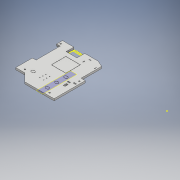
# Autodesk Inventor part: Circuit_handmainboard
Saved by Autodesk Inventor 2018.2 (Build 222227000, 227)
## iProperties
Created: 2018-02-16
Part Number: Circuit_handmainboard
Material: 一般
Document SubType Name: Modeling
Designer: sktom
Density: 1 g/cm^3
Appearance: 既定
Author: sktom
Autodesk Inventor part; units mm, degrees
ref_plane "YZ Plane" through (0, 0, 0) normal (1, 0, 0) x (0, 1, 0)
ref_plane "XZ Plane" through (0, 0, 0) normal (0, 1, 0) x (-1, 0, 0)
ref_plane "XY Plane" through (0, 0, 0) normal (0, 0, 1) x (1, 0, 0)
ref_plane "作業平面1" through (-67.9371, -16.7147, 8.5971) normal (0, 0, -1) x (1, 0, 0)
sketch "スケッチ1" plane through (-67.9371, -16.7147, 8.5971) normal (0, 0, -1) x (1, 0, 0)
  line L0 (13.1301, 23.5542) -> (-11.3844, 23.5542)
  line L1 (-11.3844, 23.5542) -> (-17.9394, 16.9992)
  line L2 (-17.9394, 16.9992) -> (-25.6445, 16.9992)
  line L3 (-25.6445, 16.9992) -> (-25.6445, 2.9992)
  line L4 (-25.6445, 2.9992) -> (-22.5935, 2.9992)
  line L5 (-22.5935, 2.9992) -> (-22.5935, -17.3653)
  line L6 (-22.5935, -17.3653) -> (-25.6833, -17.3653)
  line L7 (-25.6833, -17.3653) -> (-25.6833, -22.3653)
  line L8 (-25.6833, -22.3653) -> (4.3167, -22.3653)
  line L9 (9.5791, -2.734) -> (13.1301, -2.734)
  line L10 (13.1301, -2.734) -> (13.1301, 23.5542)
  line L11 (-25.6445, 19.5692) -> (-19.0435, 19.5692) construction
  line L12 (-25.6445, 19.5692) -> (-25.6445, 17.4992) construction
  line L13 (-25.6445, 17.4992) -> (-18.1465, 17.4992) construction
  line L14 (-18.1465, 17.4992) -> (-11.5915, 24.0542) construction
  line L15 (-11.5915, 24.0542) -> (8.4875, 24.0542) construction
  line L16 (8.4875, 24.0542) -> (8.4875, 26.1242) construction
  line L17 (8.4875, 26.1242) -> (-12.4885, 26.1242) construction
  line L18 (-12.4885, 26.1242) -> (-19.0435, 19.5692) construction
  line L19 (12.2825, 24.0542) -> (14.4905, 24.0542) construction
  line L20 (12.2825, 26.1242) -> (12.2825, 24.0542) construction
  line L21 (12.2825, 24.0542) -> (14.4905, 24.0542) construction
  line L22 (14.4905, 25.4342) -> (14.4905, 24.0542) construction
  line L23 (14.4905, 25.4342) -> (14.4905, 26.1242) construction
  line L24 (14.4905, 26.1242) -> (12.2825, 26.1242) construction
  arc A0 (18.044, 32.4032) -> (16.25, 34.1972) centre (16.25, 32.4032) ccw construction
  line L25 (14.4905, 34.1972) -> (16.25, 34.1972) construction
  line L26 (14.4905, 22.1222) -> (14.4905, 34.1972) construction
  line L27 (14.4905, 22.1222) -> (16.6625, 22.1222) construction
  spline S0 degree 3 poles (16.6625, 22.1222) (16.6025, 24.0843) (16.7566, 25.754) (17.2827, 28.3804) (17.6102, 29.4664) (18.044, 30.5621) knots 0 0 0 0 0.588904 0.588904 1.048143 1.048143 1.048143 1.048143 construction
  line L28 (18.044, 30.5621) -> (18.044, 32.4032) construction
  circle A1 centre (16.25, 32.4032) radius 0.759 construction
  circle A2 centre (6.83, 21.0542) radius 0.55 construction
  circle A3 centre (6.83, 21.0542) radius 1.25 construction
  circle A4 centre (-20.44, 14.4992) radius 1.25 construction
  line L29 (-26.4335, 26.3431) -> (-29.1935, 26.3431) construction
  line L30 (-29.1935, -10.9394) -> (-29.1935, 26.3431) construction
  line L31 (-26.4335, -10.9394) -> (-29.1935, -10.9394) construction
  line L32 (-26.4335, 26.3431) -> (-26.4335, -10.9394) construction
  line L33 (-24.0935, -8.7226) -> (-24.0935, -12.2226) construction
  circle A5 centre (-24.1833, -19.3653) radius 0.55 construction
  circle A6 centre (-24.1833, -19.3653) radius 1.25 construction
  line L34 (9.1301, -21.8653) -> (-26.1833, -21.8653) construction
  line L35 (-26.1833, -21.8653) -> (-26.1833, -22.2455) construction
  spline S1 degree 3 poles (-26.1833, -22.2455) (-26.0411, -22.8107) (-25.8944, -23.3732) (-25.7431, -23.9353) knots 0 0 0 0 1 1 1 1 construction
  line L36 (8.4752, -23.9353) -> (-25.7431, -23.9353) construction
  spline S2 degree 3 poles (8.4752, -23.9353) (8.5807, -23.5922) (8.6886, -23.2482) (8.9069, -22.5597) (9.0189, -22.2107) (9.1301, -21.8653) knots 0 0 0 0 0.496471 0.496471 1 1 1 1 construction
  circle A7 centre (11.1301, 0.266) radius 0.55 construction
  circle A8 centre (11.1301, 0.266) radius 1.25 construction
  line L37 (11.489, 24.0542) -> (11.489, 1.4634) construction
  line L38 (-1.4209, -20.0276) -> (-1.4166, -12.0276) construction
  line L39 (-1.4209, -20.0276) -> (9.5791, -20.0335) construction
  line L40 (9.5834, -12.0335) -> (9.5791, -20.0335) construction
  line L41 (-1.4166, -12.0276) -> (9.5834, -12.0335) construction
  line L42 (8.8105, 9.9742) -> (7.3105, 9.9742) construction
  line L43 (7.3105, 9.9742) -> (7.3105, 7.2742) construction
  line L44 (7.3105, 7.2742) -> (8.8105, 7.2742) construction
  line L45 (8.8105, 7.2742) -> (8.8105, 9.9742) construction
  line L46 (19.5605, 12.1242) -> (6.5605, 12.1242) construction
  line L47 (19.5605, 12.1242) -> (19.5605, 3.1242) construction
  line L48 (19.5605, 3.1242) -> (6.5605, 3.1242) construction
  line L49 (6.5605, 4.8242) -> (6.5605, 3.1242) construction
  line L50 (6.5605, 4.8242) -> (8.2605, 4.8242) construction
  line L51 (8.2605, 4.8242) -> (8.2605, 5.6242) construction
  line L52 (8.2605, 5.6242) -> (6.5605, 5.6242) construction
  line L53 (6.5605, 12.1242) -> (6.5605, 5.6242) construction
  line L54 (11.7605, 4.1242) -> (9.7605, 4.1242) construction
  line L55 (9.7605, 4.1242) -> (9.7605, 3.3242) construction
  line L56 (9.7605, 3.3242) -> (11.7605, 3.3242) construction
  line L57 (11.7605, 3.3242) -> (11.7605, 4.1242) construction
  circle A9 centre (14.5605, 10.1242) radius 0.75 construction
  circle A10 centre (14.5605, 5.1242) radius 0.75 construction
  line L58 (9.5791, -20.0335) -> (4.3167, -22.3653)
  line L59 (9.5791, -20.0335) -> (9.5791, -2.734)
  circle A11 centre (6.83, 21.0542) radius 0.55
  circle A12 centre (-20.44, 14.4992) radius 0.55
  circle A13 centre (11.1301, 0.266) radius 0.55
  circle A14 centre (-24.1833, -19.3653) radius 0.55
  point P0 (67.9371, -16.7147)
  point P1 (9.6055, 25.0467)
  dimension "d0" = 0.5
  dimension "d2" = 0.5
  dimension "d3" = 0.5
  dimension "d4" = 14
  dimension "d5" = 1.5
  dimension "d6" = 2
  dimension "d8" = 0.5
  dimension "d9" = 5
  dimension "d10" = 30
  dimension "d11" = 3
  dimension "d12" = 2
  constraints: 26 end point, 5 perpendicular, 4 centre point, 4 coincident, 4 equal radius, 3 vertical, 2 horizontal, 2 parallel, 1 vertical alignment, 2 other
  measures "d0" distance between parallel lines of L15 L0
  measures "d2" distance between parallel lines of L13 L2
  measures "d3" distance between parallel lines of L14 L1
  measures "d4" distance of L2.end L3.end
  measures "d5" distance between parallel lines of L5 L33
  measures "d6" distance from line of A5.centre L6
  measures "d8" distance between parallel lines of L7 L35
  measures "d9" distance of L6.end L7.end
  measures "d10" distance of L7.end L8.end
  measures "d11" distance from line of A7.centre L9
  measures "d12" distance from line of L10 A7.centre
extrude "押し出し1" add sketch "スケッチ1" along normal blind 1.6
sketch "スケッチ2" plane through (-67.9371, -16.7147, 8.5971) normal (0, 0, 1) x (1, 0, 0)
  line L0 (0.8793, 19.6788) -> (0.8791, 19.9788) projected
  line L1 (0.8791, 19.9788) -> (-0.7209, 19.978) projected
  line L2 (-0.7209, 19.978) -> (-0.7207, 19.678) projected
  line L3 (-0.7207, 19.678) -> (0.8793, 19.6788) projected
  line L4 (-1.5692, 16.8275) -> (-1.5683, 15.2275) projected
  line L5 (-1.5683, 15.2275) -> (-1.2683, 15.2277) projected
  line L6 (-1.2683, 15.2277) -> (-1.2692, 16.8277) projected
  line L7 (-1.2692, 16.8277) -> (-1.5692, 16.8275) projected
  line L8 (8.4317, 15.2329) -> (8.4308, 16.8329) projected
  line L9 (8.4308, 16.8329) -> (8.1308, 16.8327) projected
  line L10 (8.1308, 16.8327) -> (8.1317, 15.2327) projected
  line L11 (8.1317, 15.2327) -> (8.4317, 15.2329) projected
  line L12 (8.8105, -9.9742) -> (8.8105, -7.2742) projected
  line L13 (8.8105, -7.2742) -> (7.3105, -7.2742) projected
  line L14 (7.3105, -7.2742) -> (7.3105, -9.9742) projected
  line L15 (7.3105, -9.9742) -> (8.8105, -9.9742) projected
  line L16 (8.2605, -5.6242) -> (8.2605, -4.8242) projected
  line L17 (8.2605, -4.8242) -> (6.2605, -4.8242) projected
  line L18 (6.2605, -4.8242) -> (6.2605, -5.6242) projected
  line L19 (6.2605, -5.6242) -> (8.2605, -5.6242) projected
  line L20 (11.7605, -4.1242) -> (11.7605, -3.3242) projected
  line L21 (11.7605, -3.3242) -> (9.7605, -3.3242) projected
  line L22 (9.7605, -3.3242) -> (9.7605, -4.1242) projected
  line L23 (9.7605, -4.1242) -> (11.7605, -4.1242) projected
  line L24 (1.9385, -11.6679) -> (2.7385, -11.6675) projected
  arc A0 (2.7385, -11.6675) -> (2.7373, -9.4675) centre (2.7379, -10.5675) ccw projected
  line L25 (2.7373, -9.4675) -> (1.9373, -9.4679) projected
  arc A1 (1.9373, -9.4679) -> (1.9385, -11.6679) centre (1.9379, -10.5679) ccw projected
  line L26 (4.4375, -9.8666) -> (4.4371, -9.1666) projected
  line L27 (4.4375, -9.8666) -> (4.6375, -9.8665) projected
  line L28 (4.6375, -9.8665) -> (4.6371, -9.1665) projected
  line L29 (4.6371, -9.1665) -> (4.4371, -9.1666) projected
  line L30 (4.4386, -11.9666) -> (4.4382, -11.2666) projected
  line L31 (4.6386, -11.9665) -> (4.4386, -11.9666) projected
  line L32 (4.6382, -11.2665) -> (4.6386, -11.9665) projected
  line L33 (4.4382, -11.2666) -> (4.6382, -11.2665) projected
  line L34 (0.2382, -11.2689) -> (0.2386, -11.9689) projected
  line L35 (0.2382, -11.2689) -> (0.0382, -11.269) projected
  line L36 (0.0382, -11.269) -> (0.0386, -11.969) projected
  line L37 (0.0386, -11.969) -> (0.2386, -11.9689) projected
  line L38 (0.2371, -9.1689) -> (0.2375, -9.8689) projected
  line L39 (0.0371, -9.169) -> (0.2371, -9.1689) projected
  line L40 (0.0375, -9.869) -> (0.0371, -9.169) projected
  line L41 (0.2375, -9.8689) -> (0.0375, -9.869) projected
  line L42 (1.9343, -3.8679) -> (2.7343, -3.8675) projected
  arc A2 (2.7343, -3.8675) -> (2.7331, -1.6675) centre (2.7337, -2.7675) ccw projected
  line L43 (2.7331, -1.6675) -> (1.9331, -1.6679) projected
  arc A3 (1.9331, -1.6679) -> (1.9343, -3.8679) centre (1.9337, -2.7679) ccw projected
  line L44 (0.2329, -1.3689) -> (0.2333, -2.0689) projected
  line L45 (0.0329, -1.369) -> (0.2329, -1.3689) projected
  line L46 (0.0333, -2.069) -> (0.0329, -1.369) projected
  line L47 (0.2333, -2.0689) -> (0.0333, -2.069) projected
  line L48 (0.234, -3.4689) -> (0.2344, -4.1689) projected
  line L49 (0.234, -3.4689) -> (0.034, -3.469) projected
  line L50 (0.034, -3.469) -> (0.0344, -4.169) projected
  line L51 (0.0344, -4.169) -> (0.2344, -4.1689) projected
  line L52 (4.4333, -2.0666) -> (4.4329, -1.3666) projected
  line L53 (4.4333, -2.0666) -> (4.6333, -2.0665) projected
  line L54 (4.6333, -2.0665) -> (4.6329, -1.3665) projected
  line L55 (4.6329, -1.3665) -> (4.4329, -1.3666) projected
  line L56 (4.4344, -4.1666) -> (4.434, -3.4666) projected
  line L57 (4.6344, -4.1665) -> (4.4344, -4.1666) projected
  line L58 (4.634, -3.4665) -> (4.6344, -4.1665) projected
  line L59 (4.434, -3.4666) -> (4.634, -3.4665) projected
  line L60 (1.9427, -19.4679) -> (2.7427, -19.4675) projected
  arc A4 (2.7427, -19.4675) -> (2.7415, -17.2675) centre (2.7421, -18.3675) ccw projected
  line L61 (2.7415, -17.2675) -> (1.9415, -17.2679) projected
  arc A5 (1.9415, -17.2679) -> (1.9427, -19.4679) centre (1.9421, -18.3679) ccw projected
  line L62 (4.4417, -17.6666) -> (4.4413, -16.9666) projected
  line L63 (4.4417, -17.6666) -> (4.6417, -17.6665) projected
  line L64 (4.6417, -17.6665) -> (4.6413, -16.9665) projected
  line L65 (4.6413, -16.9665) -> (4.4413, -16.9666) projected
  line L66 (4.4428, -19.7666) -> (4.4424, -19.0666) projected
  line L67 (4.6428, -19.7665) -> (4.4428, -19.7666) projected
  line L68 (4.6424, -19.0665) -> (4.6428, -19.7665) projected
  line L69 (4.4424, -19.0666) -> (4.6424, -19.0665) projected
  line L70 (0.2413, -16.9689) -> (0.2417, -17.6689) projected
  line L71 (0.0413, -16.969) -> (0.2413, -16.9689) projected
  line L72 (0.0417, -17.669) -> (0.0413, -16.969) projected
  line L73 (0.2417, -17.6689) -> (0.0417, -17.669) projected
  line L74 (0.0424, -19.069) -> (0.0428, -19.769) projected
  line L75 (-8.248, -15.9785) -> (-4.748, -15.9766) projected
  line L76 (-8.2489, -14.4285) -> (-8.248, -15.9785) projected
  line L77 (-8.2526, -7.4785) -> (-8.2518, -9.0285) projected
  line L78 (-4.7526, -7.4766) -> (-8.2526, -7.4785) projected
  line L79 (-17.6713, -14.064) -> (-13.4713, -14.0617) projected
  line L80 (-13.4713, -14.0617) -> (-13.473, -10.8617) projected
  line L81 (-13.473, -10.8617) -> (-17.673, -10.864) projected
  line L82 (-17.673, -10.864) -> (-17.6713, -14.064) projected
  line L83 (-13.5213, -14.0117) -> (-14.3713, -14.0122) projected
  line L84 (-14.3713, -14.0122) -> (-13.5217, -13.1617) projected
  line L85 (-13.5217, -13.1617) -> (-13.5213, -14.0117) projected
  line L86 (-16.7713, -14.0135) -> (-17.6213, -14.0139) projected
  line L87 (-17.6213, -14.0139) -> (-17.6217, -13.1639) projected
  line L88 (-17.6217, -13.1639) -> (-16.7713, -14.0135) projected
  line L89 (-14.3729, -10.9122) -> (-13.523, -10.9117) projected
  line L90 (-13.523, -10.9117) -> (-13.5225, -11.7617) projected
  line L91 (-13.5225, -11.7617) -> (-14.3729, -10.9122) projected
  line L92 (-17.6229, -10.9139) -> (-16.7729, -10.9135) projected
  line L93 (-16.7729, -10.9135) -> (-17.6225, -11.7639) projected
  line L94 (-17.6225, -11.7639) -> (-17.6229, -10.9139) projected
  arc A6 (-15.9727, -11.363) -> (-15.9715, -13.563) centre (-15.9721, -12.463) ccw projected
  line L95 (-15.9727, -11.363) -> (-15.1727, -11.3626) projected
  arc A7 (-15.1715, -13.5626) -> (-15.1727, -11.3626) centre (-15.1721, -12.4626) ccw projected
  line L96 (-15.1715, -13.5626) -> (-15.9715, -13.563) projected
  line L97 (-1.5207, 1.0375) -> (-1.5262, 11.2275) projected
  line L98 (-11.7107, 1.032) -> (-1.5207, 1.0375) projected
  line L99 (-11.7162, 11.222) -> (-11.7107, 1.032) projected
  line L100 (-1.5262, 11.2275) -> (-11.7162, 11.222) projected
  line L101 (-0.5201, 0.0381) -> (-12.7101, 0.0315) projected
  line L102 (-0.5267, 12.2281) -> (-0.5201, 0.0381) projected
  line L103 (-12.7167, 12.2215) -> (-0.5267, 12.2281) projected
  line L104 (-12.7101, 0.0315) -> (-12.7167, 12.2215) projected
  point P0 (67.9371, 16.7147)
sketch "スケッチ3" plane through (-67.9371, -16.7147, 6.9971) normal (0, 0, -1) x (-1, 0, 0)
  line L0 (19.1277, -4.5638) -> (3.8877, -4.5555) projected
  line L1 (19.1414, 20.8362) -> (19.1277, -4.5638) projected
  line L2 (3.9014, 20.8445) -> (19.1414, 20.8362) projected
  line L3 (3.8877, -4.5555) -> (3.9014, 20.8445) projected
  circle A0 centre (8.9697, -0.7483) radius 0.51 projected
  circle A1 centre (11.5097, -0.7497) radius 0.51 projected
  circle A2 centre (14.0497, -0.751) radius 0.51 projected
  circle A3 centre (5.1597, -0.7462) radius 0.51 projected
  circle A4 centre (5.1625, 4.3338) radius 0.51 projected
  circle A5 centre (5.1652, 9.4138) radius 0.51 projected
  circle A6 centre (5.1679, 14.4938) radius 0.51 projected
  circle A7 centre (5.1707, 19.5738) radius 0.51 projected
  circle A8 centre (17.8597, -0.7531) radius 0.51 projected
  circle A9 centre (17.8625, 4.3269) radius 0.51 projected
  circle A10 centre (17.8652, 9.4069) radius 0.51 projected
  circle A11 centre (17.8679, 14.4869) radius 0.51 projected
  circle A12 centre (17.8707, 19.5669) radius 0.51 projected
  circle A13 centre (17.8693, 17.0269) radius 0.51 projected
  circle A14 centre (17.8666, 11.9469) radius 0.51 projected
  circle A15 centre (17.8638, 6.8669) radius 0.51 projected
  circle A16 centre (17.8611, 1.7869) radius 0.51 projected
  circle A17 centre (17.8584, -3.2931) radius 0.51 projected
  circle A18 centre (5.1693, 17.0338) radius 0.51 projected
  circle A19 centre (5.1666, 11.9538) radius 0.51 projected
  circle A20 centre (5.1638, 6.8738) radius 0.51 projected
  circle A21 centre (5.1611, 1.7938) radius 0.51 projected
  circle A22 centre (5.1584, -3.2862) radius 0.51 projected
  circle A23 centre (14.0484, -3.291) radius 0.51 projected
  circle A24 centre (11.5084, -3.2897) radius 0.51 projected
  circle A25 centre (8.9684, -3.2883) radius 0.51 projected
  line L4 (20.6136, 6.3654) -> (20.6141, 7.3654) projected
  line L5 (20.6141, 7.3654) -> (19.1141, 7.3662) projected
  line L6 (19.1136, 6.3662) -> (19.1141, 7.3662) projected
  line L7 (19.1136, 6.3662) -> (20.6136, 6.3654) projected
  line L8 (20.6163, 11.4454) -> (20.6168, 12.4454) projected
  line L9 (20.6168, 12.4454) -> (19.1168, 12.4462) projected
  line L10 (19.1163, 11.4462) -> (19.1168, 12.4462) projected
  line L11 (19.1163, 11.4462) -> (20.6163, 11.4454) projected
  line L12 (20.619, 16.5254) -> (20.6196, 17.5254) projected
  line L13 (20.6196, 17.5254) -> (19.1196, 17.5262) projected
  line L14 (19.119, 16.5262) -> (19.1196, 17.5262) projected
  line L15 (19.119, 16.5262) -> (20.619, 16.5254) projected
  line L16 (19.1108, 1.2863) -> (20.6108, 1.2854) projected
  line L17 (20.6108, 1.2854) -> (20.6114, 2.2854) projected
  line L18 (20.6114, 2.2854) -> (19.1114, 2.2862) projected
  line L19 (19.1108, 1.2863) -> (19.1114, 2.2862) projected
  line L20 (19.1108, 1.2863) -> (20.6108, 1.2854) projected
  line L21 (20.6081, -3.7946) -> (20.6086, -2.7946) projected
  line L22 (20.6086, -2.7946) -> (19.1086, -2.7937) projected
  line L23 (19.1081, -3.7937) -> (19.1086, -2.7937) projected
  line L24 (19.1081, -3.7937) -> (20.6081, -3.7946) projected
  line L25 (2.4095, -1.2447) -> (2.41, -0.2447) projected
  line L26 (3.9095, -1.2456) -> (2.4095, -1.2447) projected
  line L27 (3.91, -0.2456) -> (3.9095, -1.2456) projected
  line L28 (2.41, -0.2447) -> (3.91, -0.2456) projected
  line L29 (2.4122, 3.8353) -> (2.4127, 4.8353) projected
  line L30 (3.9122, 3.8344) -> (2.4122, 3.8353) projected
  line L31 (3.9127, 4.8344) -> (3.9122, 3.8344) projected
  line L32 (2.4127, 4.8353) -> (3.9127, 4.8344) projected
  line L33 (2.4149, 8.9153) -> (2.4155, 9.9153) projected
  line L34 (3.9149, 8.9144) -> (2.4149, 8.9153) projected
  line L35 (3.9155, 9.9144) -> (3.9149, 8.9144) projected
  line L36 (2.4155, 9.9153) -> (3.9155, 9.9144) projected
  line L37 (2.4177, 13.9953) -> (2.4182, 14.9953) projected
  line L38 (3.9177, 13.9944) -> (2.4177, 13.9953) projected
  line L39 (3.9182, 14.9944) -> (3.9177, 13.9944) projected
  line L40 (2.4182, 14.9953) -> (3.9182, 14.9944) projected
  line L41 (2.4204, 19.0752) -> (2.4209, 20.0752) projected
  line L42 (3.9204, 19.0744) -> (2.4204, 19.0752) projected
  line L43 (3.9209, 20.0744) -> (3.9204, 19.0744) projected
  line L44 (2.4209, 20.0752) -> (3.9209, 20.0744) projected
  circle A26 centre (8.1017, -9.2284) radius 0.25 projected
  circle A27 centre (8.1003, -11.7284) radius 0.25 projected
  circle A28 centre (8.099, -14.2284) radius 0.25 projected
  circle A29 centre (4.899, -14.2266) radius 0.25 projected
  circle A30 centre (4.9003, -11.7266) radius 0.25 projected
  circle A31 centre (4.9017, -9.2266) radius 0.25 projected
  line L45 (-7.3839, 11.0323) -> (-6.0839, 11.0316) projected
  line L46 (-7.3839, 11.0323) -> (-7.3854, 8.2323) projected
  line L47 (-7.3854, 8.2323) -> (-6.0854, 8.2316) projected
  line L48 (-6.0839, 11.0316) -> (-6.0854, 8.2316) projected
  line L49 (-0.1839, 11.0284) -> (1.1161, 11.0277) projected
  line L50 (-0.1839, 11.0284) -> (-0.1854, 8.2284) projected
  line L51 (-0.1854, 8.2284) -> (1.1146, 8.2277) projected
  line L52 (1.1161, 11.0277) -> (1.1146, 8.2277) projected
  line L53 (-1.7259, 7.4263) -> (-1.7261, 6.9293) projected
  line L54 (-1.7259, 7.4263) -> (-2.0459, 7.4264) projected
  line L55 (-2.0459, 7.4264) -> (-2.0461, 6.9294) projected
  line L56 (-1.7261, 6.9293) -> (-2.0461, 6.9294) projected
  line L57 (-2.9759, 7.4269) -> (-2.9761, 6.9299) projected
  line L58 (-2.9759, 7.4269) -> (-3.2959, 7.4271) projected
  line L59 (-3.2959, 7.4271) -> (-3.2961, 6.9301) projected
  line L60 (-2.9761, 6.9299) -> (-3.2961, 6.9301) projected
  line L61 (-4.2259, 7.4276) -> (-4.2261, 6.9306) projected
  line L62 (-4.2259, 7.4276) -> (-4.5459, 7.4278) projected
  line L63 (-4.5459, 7.4278) -> (-4.5461, 6.9308) projected
  line L64 (-4.2261, 6.9306) -> (-4.5461, 6.9308) projected
  line L65 (-0.1867, 5.8284) -> (1.1133, 5.8277) projected
  line L66 (-0.1867, 5.8284) -> (-0.1882, 3.0284) projected
  line L67 (-0.1882, 3.0284) -> (1.1118, 3.0277) projected
  line L68 (1.1133, 5.8277) -> (1.1118, 3.0277) projected
  line L69 (-7.3867, 5.8323) -> (-6.0867, 5.8316) projected
  line L70 (-7.3867, 5.8323) -> (-7.3882, 3.0323) projected
  line L71 (-7.3882, 3.0323) -> (-6.0882, 3.0316) projected
  line L72 (-6.0867, 5.8316) -> (-6.0882, 3.0316) projected
  line L73 (-4.2287, 2.2276) -> (-4.2289, 1.7306) projected
  line L74 (-4.2287, 2.2276) -> (-4.5487, 2.2278) projected
  line L75 (-4.5487, 2.2278) -> (-4.5489, 1.7308) projected
  line L76 (-4.2289, 1.7306) -> (-4.5489, 1.7308) projected
  line L77 (-2.9787, 2.2269) -> (-2.9789, 1.7299) projected
  line L78 (-2.9787, 2.2269) -> (-3.2987, 2.2271) projected
  line L79 (-3.2987, 2.2271) -> (-3.2989, 1.7301) projected
  line L80 (-2.9789, 1.7299) -> (-3.2989, 1.7301) projected
  line L81 (-1.7287, 2.2263) -> (-1.7289, 1.7293) projected
  line L82 (-1.7287, 2.2263) -> (-2.0487, 2.2264) projected
  line L83 (-2.0487, 2.2264) -> (-2.0489, 1.7294) projected
  line L84 (-1.7289, 1.7293) -> (-2.0489, 1.7294) projected
  line L85 (25.465, -4.935) -> (25.4643, -6.235) projected
  line L86 (25.465, -4.935) -> (22.665, -4.9335) projected
  line L87 (22.665, -4.9335) -> (22.6643, -6.2335) projected
  line L88 (25.4643, -6.235) -> (22.6643, -6.2335) projected
  line L89 (21.8603, -8.093) -> (21.3633, -8.0928) projected
  line L90 (21.8603, -8.093) -> (21.8604, -7.773) projected
  line L91 (21.8604, -7.773) -> (21.3634, -7.7728) projected
  line L92 (21.3633, -8.0928) -> (21.3634, -7.7728) projected
  line L93 (21.8596, -9.343) -> (21.3626, -9.3428) projected
  line L94 (21.8596, -9.343) -> (21.8598, -9.023) projected
  line L95 (21.8598, -9.023) -> (21.3628, -9.0228) projected
  line L96 (21.3626, -9.3428) -> (21.3628, -9.0228) projected
  line L97 (21.8589, -10.593) -> (21.3619, -10.5928) projected
  line L98 (21.8589, -10.593) -> (21.8591, -10.273) projected
  line L99 (21.8591, -10.273) -> (21.3621, -10.2728) projected
  line L100 (21.3619, -10.5928) -> (21.3621, -10.2728) projected
  line L101 (25.4611, -12.135) -> (25.4604, -13.435) projected
  line L102 (25.4611, -12.135) -> (22.6611, -12.1335) projected
  line L103 (22.6611, -12.1335) -> (22.6604, -13.4335) projected
  line L104 (25.4604, -13.435) -> (22.6604, -13.4335) projected
  line L105 (17.869, 16.5269) -> (17.8696, 17.5269) projected
  line L106 (17.8696, 17.5269) -> (20.6196, 17.5254) projected
  line L107 (20.6196, 17.5254) -> (20.619, 16.5254) projected
  line L108 (20.619, 16.5254) -> (17.869, 16.5269) projected
  line L109 (17.8709, 20.0669) -> (17.8704, 19.0669) projected
  line L110 (17.8704, 19.0669) -> (15.1204, 19.0684) projected
  line L111 (15.1204, 19.0684) -> (15.1209, 20.0684) projected
  line L112 (15.1209, 20.0684) -> (17.8709, 20.0669) projected
  line L113 (16.6177, 13.9876) -> (15.1177, 13.9884) projected
  line L114 (17.8682, 14.9869) -> (17.8677, 13.9869) projected
  line L115 (17.8677, 13.9869) -> (15.1177, 13.9884) projected
  line L116 (15.1177, 13.9884) -> (15.1182, 14.9884) projected
  line L117 (15.1182, 14.9884) -> (17.8682, 14.9869) projected
  line L118 (17.8663, 11.4469) -> (17.8668, 12.4469) projected
  line L119 (17.8668, 12.4469) -> (20.6168, 12.4454) projected
  line L120 (20.6168, 12.4454) -> (20.6163, 11.4454) projected
  line L121 (20.6163, 11.4454) -> (17.8663, 11.4469) projected
  line L122 (17.8655, 9.9069) -> (17.8649, 8.9069) projected
  line L123 (17.8649, 8.9069) -> (15.1149, 8.9084) projected
  line L124 (15.1149, 8.9084) -> (15.1155, 9.9084) projected
  line L125 (15.1155, 9.9084) -> (17.8655, 9.9069) projected
  line L126 (17.8636, 6.3669) -> (17.8641, 7.3669) projected
  line L127 (17.8641, 7.3669) -> (20.6141, 7.3654) projected
  line L128 (20.6141, 7.3654) -> (20.6136, 6.3654) projected
  line L129 (20.6136, 6.3654) -> (17.8636, 6.3669) projected
  line L130 (17.8627, 4.8269) -> (17.8622, 3.8269) projected
  line L131 (17.8622, 3.8269) -> (15.1122, 3.8284) projected
  line L132 (15.1122, 3.8284) -> (15.1127, 4.8284) projected
  line L133 (15.1127, 4.8284) -> (17.8627, 4.8269) projected
  line L134 (17.8608, 1.2869) -> (17.8614, 2.2869) projected
  line L135 (17.8614, 2.2869) -> (20.6114, 2.2854) projected
  line L136 (20.6114, 2.2854) -> (20.6108, 1.2854) projected
  line L137 (20.6108, 1.2854) -> (17.8608, 1.2869) projected
  line L138 (17.86, -0.2531) -> (17.8595, -1.2531) projected
  line L139 (17.8595, -1.2531) -> (15.1095, -1.2516) projected
  line L140 (15.1095, -1.2516) -> (15.11, -0.2516) projected
  line L141 (15.11, -0.2516) -> (17.86, -0.2531) projected
  line L142 (17.8581, -3.7931) -> (17.8586, -2.7931) projected
  line L143 (17.8586, -2.7931) -> (20.6086, -2.7946) projected
  line L144 (20.6086, -2.7946) -> (20.6081, -3.7946) projected
  line L145 (20.6081, -3.7946) -> (17.8581, -3.7931) projected
  line L146 (5.1581, -3.7862) -> (5.1586, -2.7862) projected
  line L147 (5.1586, -2.7862) -> (7.9086, -2.7877) projected
  line L148 (7.9086, -2.7877) -> (7.9081, -3.7877) projected
  line L149 (7.9081, -3.7877) -> (5.1581, -3.7862) projected
  line L150 (5.16, -0.2462) -> (5.1595, -1.2462) projected
  line L151 (5.1595, -1.2462) -> (2.4095, -1.2447) projected
  line L152 (2.4095, -1.2447) -> (2.41, -0.2447) projected
  line L153 (2.41, -0.2447) -> (5.16, -0.2462) projected
  line L154 (5.1608, 1.2938) -> (5.1614, 2.2938) projected
  line L155 (5.1614, 2.2938) -> (7.9114, 2.2923) projected
  line L156 (7.9114, 2.2923) -> (7.9108, 1.2923) projected
  line L157 (7.9108, 1.2923) -> (5.1608, 1.2938) projected
  line L158 (5.1709, 20.0738) -> (5.1704, 19.0738) projected
  line L159 (5.1704, 19.0738) -> (2.4204, 19.0752) projected
  line L160 (2.4204, 19.0752) -> (2.4209, 20.0752) projected
  line L161 (2.4209, 20.0752) -> (5.1709, 20.0738) projected
  line L162 (5.169, 16.5338) -> (5.1696, 17.5338) projected
  line L163 (5.1696, 17.5338) -> (7.9196, 17.5323) projected
  line L164 (7.9196, 17.5323) -> (7.919, 16.5323) projected
  line L165 (7.919, 16.5323) -> (5.169, 16.5338) projected
  line L166 (5.1682, 14.9938) -> (5.1677, 13.9938) projected
  line L167 (5.1677, 13.9938) -> (2.4177, 13.9953) projected
  line L168 (2.4177, 13.9953) -> (2.4182, 14.9953) projected
  line L169 (2.4182, 14.9953) -> (5.1682, 14.9938) projected
  line L170 (5.1663, 11.4538) -> (5.1668, 12.4538) projected
  line L171 (5.1668, 12.4538) -> (7.9168, 12.4523) projected
  line L172 (7.9168, 12.4523) -> (7.9163, 11.4523) projected
  line L173 (7.9163, 11.4523) -> (5.1663, 11.4538) projected
  line L174 (5.1655, 9.9138) -> (5.1649, 8.9138) projected
  line L175 (5.1649, 8.9138) -> (2.4149, 8.9153) projected
  line L176 (2.4149, 8.9153) -> (2.4155, 9.9153) projected
  line L177 (2.4155, 9.9153) -> (5.1655, 9.9138) projected
  point P0 (-67.9371, 16.7147)
extrude "押し出し2" cut sketch "スケッチ2" against normal up to next contours L3 L2 L1 L0 | L7 L6 L5 L4 | L11 L10 L9 L8
sketch "スケッチ4" plane through (-67.9371, -16.7147, 8.5971) normal (0, 0, 1) x (1, 0, 0)
  line L0 (7.3105, -7.2742) -> (7.3105, -9.9742) projected
  line L1 (6.2605, -4.8242) -> (6.2605, -5.6242) projected
  line L2 (9.7605, -3.3242) -> (9.7605, -4.1242) projected
  line L3 (8.8105, -9.9742) -> (8.8105, -7.2742) projected
  line L4 (8.2605, -5.6242) -> (8.2605, -4.8242) projected
  line L5 (11.7605, -4.1242) -> (11.7605, -3.3242) projected
  line L6 (7.3105, -9.9742) -> (8.8105, -9.9742)
  line L7 (8.8105, -9.9742) -> (8.8105, -7.2742)
  line L8 (8.8105, -7.2742) -> (7.3105, -7.2742)
  line L9 (7.3105, -7.2742) -> (7.3105, -9.9742)
  line L10 (6.2605, -5.6242) -> (8.2605, -5.6242)
  line L11 (8.2605, -5.6242) -> (8.2605, -4.8242)
  line L12 (8.2605, -4.8242) -> (6.2605, -4.8242)
  line L13 (6.2605, -4.8242) -> (6.2605, -5.6242)
  line L14 (9.7605, -4.1242) -> (11.7605, -4.1242)
  line L15 (11.7605, -4.1242) -> (11.7605, -3.3242)
  line L16 (11.7605, -3.3242) -> (9.7605, -3.3242)
  line L17 (9.7605, -3.3242) -> (9.7605, -4.1242)
  point P0 (67.9371, 16.7147)
  constraints: 24 end point, 6 parallel, 3 horizontal, 3 perpendicular
extrude "押し出し3" cut sketch "スケッチ4" against normal blind 1.6
sketch "スケッチ5" plane through (-67.9371, -16.7147, 8.5971) normal (0, 0, 1) x (1, 0, 0)
  arc A0 (1.9331, -1.6679) -> (1.9343, -3.8679) centre (1.9337, -2.7679) ccw projected
  line L0 (2.7331, -1.6675) -> (1.9331, -1.6679) projected
  arc A1 (2.7343, -3.8675) -> (2.7331, -1.6675) centre (2.7337, -2.7675) ccw projected
  line L1 (1.9343, -3.8679) -> (2.7343, -3.8675) projected
  line L2 (2.7373, -9.4675) -> (1.9373, -9.4679) projected
  arc A2 (1.9373, -9.4679) -> (1.9385, -11.6679) centre (1.9379, -10.5679) ccw projected
  line L3 (1.9385, -11.6679) -> (2.7385, -11.6675) projected
  arc A3 (2.7385, -11.6675) -> (2.7373, -9.4675) centre (2.7379, -10.5675) ccw projected
  line L4 (2.7415, -17.2675) -> (1.9415, -17.2679) projected
  arc A4 (1.9415, -17.2679) -> (1.9427, -19.4679) centre (1.9421, -18.3679) ccw projected
  line L5 (1.9427, -19.4679) -> (2.7427, -19.4675) projected
  arc A5 (2.7427, -19.4675) -> (2.7415, -17.2675) centre (2.7421, -18.3675) ccw projected
  arc A6 (-15.9727, -11.363) -> (-15.9715, -13.563) centre (-15.9721, -12.463) ccw projected
  line L6 (-15.9727, -11.363) -> (-15.1727, -11.3626) projected
  arc A7 (-15.1715, -13.5626) -> (-15.1727, -11.3626) centre (-15.1721, -12.4626) ccw projected
  line L7 (-15.1715, -13.5626) -> (-15.9715, -13.563) projected
  point P0 (67.9371, 16.7147)
extrude "押し出し4" cut sketch "スケッチ5" against normal blind 0.1
sketch "スケッチ6" plane through (-67.9371, -16.7147, 8.5971) normal (0, 0, 1) x (1, 0, 0)
  line L0 (-12.7101, 0.0315) -> (-12.7167, 12.2215) projected
  line L1 (-12.7167, 12.2215) -> (-0.5267, 12.2281) projected
  line L2 (-0.5267, 12.2281) -> (-0.5201, 0.0381) projected
  line L3 (-0.5201, 0.0381) -> (-12.7101, 0.0315) projected
  point P0 (67.9371, 16.7147)
extrude "押し出し5" cut sketch "スケッチ6" against normal blind 0.1
sketch "スケッチ7" plane through (-67.9371, -16.7147, 6.9971) normal (0, 0, -1) x (-1, 0, 0)
  circle A0 centre (4.899, -14.2266) radius 0.25 projected
  circle A1 centre (8.099, -14.2284) radius 0.25 projected
  circle A2 centre (8.1003, -11.7284) radius 0.25 projected
  circle A3 centre (4.9003, -11.7266) radius 0.25 projected
  circle A4 centre (4.9017, -9.2266) radius 0.25 projected
  circle A5 centre (8.1017, -9.2284) radius 0.25 projected
  point P0 (-67.9371, 16.7147)
extrude "押し出し6" cut sketch "スケッチ3" against normal up to next contours A26 | A27 | A28 | A29 | A30 | A31
sketch "スケッチ8" plane through (-67.9371, -16.7147, 6.9971) normal (0, 0, -1) x (-1, 0, 0)
  line L0 (22.665, -4.9335) -> (22.6643, -6.2335) projected
  line L1 (25.4643, -6.235) -> (22.6643, -6.2335) projected
  line L2 (25.465, -4.935) -> (22.665, -4.9335) projected
  line L3 (25.465, -4.935) -> (25.4643, -6.235) projected
  line L4 (25.4611, -12.135) -> (22.6611, -12.1335) projected
  line L5 (22.6611, -12.1335) -> (22.6604, -13.4335) projected
  line L6 (25.4604, -13.435) -> (22.6604, -13.4335) projected
  line L7 (25.4611, -12.135) -> (25.4604, -13.435) projected
  line L8 (21.8591, -10.273) -> (21.3621, -10.2728) projected
  line L9 (21.3619, -10.5928) -> (21.3621, -10.2728) projected
  line L10 (21.8589, -10.593) -> (21.3619, -10.5928) projected
  line L11 (21.8589, -10.593) -> (21.8591, -10.273) projected
  line L12 (21.3626, -9.3428) -> (21.3628, -9.0228) projected
  line L13 (21.8596, -9.343) -> (21.3626, -9.3428) projected
  line L14 (21.8598, -9.023) -> (21.3628, -9.0228) projected
  line L15 (21.8596, -9.343) -> (21.8598, -9.023) projected
  line L16 (21.8603, -8.093) -> (21.3633, -8.0928) projected
  line L17 (21.3633, -8.0928) -> (21.3634, -7.7728) projected
  line L18 (21.8604, -7.773) -> (21.3634, -7.7728) projected
  line L19 (21.8603, -8.093) -> (21.8604, -7.773) projected
  line L20 (-7.3867, 5.8323) -> (-6.0867, 5.8316) projected
  line L21 (-7.3867, 5.8323) -> (-7.3882, 3.0323) projected
  line L22 (-7.3882, 3.0323) -> (-6.0882, 3.0316) projected
  line L23 (-6.0867, 5.8316) -> (-6.0882, 3.0316) projected
  line L24 (-0.1867, 5.8284) -> (-0.1882, 3.0284) projected
  line L25 (-0.1882, 3.0284) -> (1.1118, 3.0277) projected
  line L26 (1.1133, 5.8277) -> (1.1118, 3.0277) projected
  line L27 (-0.1867, 5.8284) -> (1.1133, 5.8277) projected
  line L28 (-1.7287, 2.2263) -> (-1.7289, 1.7293) projected
  line L29 (-1.7287, 2.2263) -> (-2.0487, 2.2264) projected
  line L30 (-2.0487, 2.2264) -> (-2.0489, 1.7294) projected
  line L31 (-1.7289, 1.7293) -> (-2.0489, 1.7294) projected
  line L32 (-2.9789, 1.7299) -> (-3.2989, 1.7301) projected
  line L33 (-2.9787, 2.2269) -> (-2.9789, 1.7299) projected
  line L34 (-2.9787, 2.2269) -> (-3.2987, 2.2271) projected
  line L35 (-3.2987, 2.2271) -> (-3.2989, 1.7301) projected
  line L36 (-4.2287, 2.2276) -> (-4.2289, 1.7306) projected
  line L37 (-4.5487, 2.2278) -> (-4.5489, 1.7308) projected
  line L38 (-4.2287, 2.2276) -> (-4.5487, 2.2278) projected
  line L39 (-4.2289, 1.7306) -> (-4.5489, 1.7308) projected
  line L40 (-7.3854, 8.2323) -> (-6.0854, 8.2316) projected
  line L41 (-6.0839, 11.0316) -> (-6.0854, 8.2316) projected
  line L42 (-7.3839, 11.0323) -> (-6.0839, 11.0316) projected
  line L43 (-7.3839, 11.0323) -> (-7.3854, 8.2323) projected
  line L44 (-4.5459, 7.4278) -> (-4.5461, 6.9308) projected
  line L45 (-4.2259, 7.4276) -> (-4.5459, 7.4278) projected
  line L46 (-4.2259, 7.4276) -> (-4.2261, 6.9306) projected
  line L47 (-4.2261, 6.9306) -> (-4.5461, 6.9308) projected
  line L48 (-3.2959, 7.4271) -> (-3.2961, 6.9301) projected
  line L49 (-2.9759, 7.4269) -> (-3.2959, 7.4271) projected
  line L50 (-2.9759, 7.4269) -> (-2.9761, 6.9299) projected
  circle A0 centre (4.9003, -11.7266) radius 0.25 projected
  circle A1 centre (8.099, -14.2284) radius 0.25 projected
  circle A2 centre (8.1017, -9.2284) radius 0.25 projected
  circle A3 centre (8.1003, -11.7284) radius 0.25 projected
  circle A4 centre (4.899, -14.2266) radius 0.25 projected
  circle A5 centre (4.9017, -9.2266) radius 0.25 projected
  line L51 (-11.7605, -4.1242) -> (-11.7605, -3.3242) projected
  line L52 (-11.7605, -3.3242) -> (-9.7605, -3.3242) projected
  line L53 (-9.7605, -3.3242) -> (-9.7605, -4.1242) projected
  line L54 (-9.7605, -4.1242) -> (-11.7605, -4.1242) projected
  line L55 (-8.2605, -5.6242) -> (-8.2605, -4.8242) projected
  line L56 (-8.2605, -4.8242) -> (-6.2605, -4.8242) projected
  line L57 (-6.2605, -4.8242) -> (-6.2605, -5.6242) projected
  line L58 (-6.2605, -5.6242) -> (-8.2605, -5.6242) projected
  line L59 (-8.8105, -9.9742) -> (-8.8105, -7.2742) projected
  line L60 (-8.8105, -7.2742) -> (-7.3105, -7.2742) projected
  line L61 (-7.3105, -7.2742) -> (-7.3105, -9.9742) projected
  line L62 (-7.3105, -9.9742) -> (-8.8105, -9.9742) projected
  line L63 (1.5683, 15.2275) -> (1.2683, 15.2277) projected
  line L64 (1.2683, 15.2277) -> (1.2692, 16.8277) projected
  line L65 (1.2692, 16.8277) -> (1.5692, 16.8275) projected
  line L66 (1.5692, 16.8275) -> (1.5683, 15.2275) projected
  line L67 (-0.8791, 19.9788) -> (0.7209, 19.978) projected
  line L68 (0.7209, 19.978) -> (0.7207, 19.678) projected
  line L69 (0.7207, 19.678) -> (-0.8793, 19.6788) projected
  line L70 (-0.8793, 19.6788) -> (-0.8791, 19.9788) projected
  line L71 (-8.4308, 16.8329) -> (-8.1308, 16.8327) projected
  line L72 (-8.1308, 16.8327) -> (-8.1317, 15.2327) projected
  line L73 (-8.1317, 15.2327) -> (-8.4317, 15.2329) projected
  line L74 (-8.4317, 15.2329) -> (-8.4308, 16.8329) projected
  circle A6 centre (24.1833, 19.3653) radius 0.55 projected
  circle A7 centre (-11.1301, -0.266) radius 0.55 projected
  circle A8 centre (20.44, -14.4992) radius 0.55 projected
  circle A9 centre (-6.83, -21.0542) radius 0.55 projected
  line L75 (-13.1301, -23.5542) -> (11.3844, -23.5542) projected
  line L76 (11.3844, -23.5542) -> (17.9394, -16.9992) projected
  line L77 (17.9394, -16.9992) -> (25.6445, -16.9992) projected
  line L78 (25.6445, -16.9992) -> (25.6445, -2.9992) projected
  line L79 (25.6445, -2.9992) -> (22.5935, -2.9992) projected
  line L80 (22.5935, -2.9992) -> (22.5935, 17.3653) projected
  line L81 (22.5935, 17.3653) -> (25.6833, 17.3653) projected
  line L82 (25.6833, 17.3653) -> (25.6833, 22.3653) projected
  line L83 (25.6833, 22.3653) -> (-4.3167, 22.3653) projected
  line L84 (-4.3167, 22.3653) -> (-9.5791, 20.0335) projected
  line L85 (-9.5791, 20.0335) -> (-9.5791, 2.734) projected
  line L86 (-9.5791, 2.734) -> (-13.1301, 2.734) projected
  line L87 (-13.1301, 2.734) -> (-13.1301, -23.5542) projected
  line L88 (-2.9761, 6.9299) -> (-3.2961, 6.9301) projected
  line L89 (-2.0459, 7.4264) -> (-2.0461, 6.9294) projected
  line L90 (-1.7259, 7.4263) -> (-2.0459, 7.4264) projected
  line L91 (-1.7259, 7.4263) -> (-1.7261, 6.9293) projected
  line L92 (-1.7261, 6.9293) -> (-2.0461, 6.9294) projected
  line L93 (-0.1854, 8.2284) -> (1.1146, 8.2277) projected
  line L94 (-0.1839, 11.0284) -> (-0.1854, 8.2284) projected
  line L95 (-0.1839, 11.0284) -> (1.1161, 11.0277) projected
  line L96 (1.1161, 11.0277) -> (1.1146, 8.2277) projected
  point P0 (-67.9371, 16.7147)
extrude "押し出し7" cut sketch "スケッチ8" against normal blind 0.1 contours L2 L3 L1 L0 | L7 L6 L5 L4 | L11 L10 L9 L8 | L16 L17 L18 L19 | L20 L23 L22 L21 | L27 L26 L25 L24 | L28 L31 L30 L29 | L36 L39 L37 L38 | L43 L42 L41 L40 | L45 L46 L47 L44 | L90 L91 L92 L89 | L94 L95 L96 L93
sketch "スケッチ9" plane through (-67.9371, -16.7147, 6.9971) normal (0, 0, -1) x (-1, 0, 0)
  line L0 (3.8877, -4.5555) -> (3.9014, 20.8445) projected
  line L1 (19.1277, -4.5638) -> (3.8877, -4.5555) projected
  line L2 (19.1414, 20.8362) -> (19.1277, -4.5638) projected
  line L3 (3.9014, 20.8445) -> (19.1414, 20.8362) projected
  circle A0 centre (5.1693, 17.0338) radius 0.51 projected
  circle A1 centre (5.1707, 19.5738) radius 0.51 projected
  circle A2 centre (5.1679, 14.4938) radius 0.51 projected
  circle A3 centre (5.1666, 11.9538) radius 0.51 projected
  circle A4 centre (5.1638, 6.8738) radius 0.51 projected
  circle A5 centre (5.1625, 4.3338) radius 0.51 projected
  circle A6 centre (5.1611, 1.7938) radius 0.51 projected
  circle A7 centre (5.1597, -0.7462) radius 0.51 projected
  circle A8 centre (5.1584, -3.2862) radius 0.51 projected
  circle A9 centre (17.8584, -3.2931) radius 0.51 projected
  circle A10 centre (17.8597, -0.7531) radius 0.51 projected
  circle A11 centre (17.8625, 4.3269) radius 0.51 projected
  circle A12 centre (17.8638, 6.8669) radius 0.51 projected
  circle A13 centre (17.8652, 9.4069) radius 0.51 projected
  circle A14 centre (17.8666, 11.9469) radius 0.51 projected
  circle A15 centre (17.8679, 14.4869) radius 0.51 projected
  circle A16 centre (17.8693, 17.0269) radius 0.51 projected
  circle A17 centre (17.8707, 19.5669) radius 0.51 projected
  point P0 (-67.9371, 16.7147)
extrude "押し出し8" cut sketch "スケッチ9" against normal blind 0.1
sketch "スケッチ10" plane through (-67.9371, -16.7147, 6.9971) normal (0, 0, -1) x (-1, 0, 0)
  line L0 (7.4714, 20.8425) -> (15.5714, 20.8382) projected
  line L1 (15.572, 21.9382) -> (15.5714, 20.8382) projected
  line L2 (7.472, 21.9425) -> (15.572, 21.9382) projected
  line L3 (7.4714, 20.8425) -> (7.472, 21.9425) projected
  line L4 (15.5689, 16.3382) -> (7.4689, 16.3425) projected
  line L5 (7.4689, 16.3425) -> (7.472, 21.9425) projected
  line L6 (7.472, 21.9425) -> (15.572, 21.9382) projected
  line L7 (15.572, 21.9382) -> (15.5689, 16.3382) projected
  point P0 (-67.9371, 16.7147)
sketch "スケッチ11" plane through (-67.9371, -16.7147, 6.9971) normal (0, 0, -1) x (-1, 0, 0)
  line L0 (25.6833, 22.3653) -> (-4.3167, 22.3653) construction
  line L1 (6.9315, 22.3653) -> (17.3597, 22.3653) construction
  line L2 (17.3597, 22.3653) -> (17.3597, 14.3499) construction
  line L3 (17.3597, 14.3499) -> (6.9315, 14.3499) construction
  line L4 (6.9315, 14.3499) -> (6.9315, 22.3653) construction
  line L5 (7.4714, 20.8425) -> (7.4689, 16.3425) construction
  line L6 (7.4689, 16.3425) -> (15.5689, 16.3382) construction
  line L7 (15.5689, 16.3382) -> (15.5714, 20.8382) construction
  point P0 (-67.9371, 16.7147)
  constraints: 8 end point, 2 parallel, 1 horizontal, 1 perpendicular, 1 point on line
sketch "スケッチ12" plane through (-67.9371, -16.7147, 6.9971) normal (0, 0, -1) x (-1, 0, 0)
  line L0 (25.6833, 22.3653) -> (-4.3167, 22.3653) projected
  line L1 (16.0689, 15.8425) -> (6.9689, 15.8425)
  line L2 (6.9689, 15.8425) -> (6.9689, 22.3653)
  line L3 (6.9689, 22.3653) -> (16.0689, 22.3653)
  line L4 (16.0689, 22.3653) -> (16.0689, 15.8425)
  line L5 (15.5689, 16.3382) -> (7.4689, 16.3425) projected
  line L6 (15.572, 21.9382) -> (15.5689, 16.3382) projected
  line L7 (7.4689, 16.3425) -> (7.472, 21.9425) projected
  point P0 (-67.9371, 16.7147)
  dimension "d30" = 0.5
  dimension "d31" = 0.5
  dimension "d32" = 0.5
  constraints: 8 end point, 2 parallel, 1 horizontal, 1 perpendicular, 1 point on line
  measures "d30" distance from line of L5.end L1
  measures "d31" distance from line of L5.end L2
  measures "d32" distance from line of L5.start L4
extrude "押し出し9" cut sketch "スケッチ12" against normal up to next
